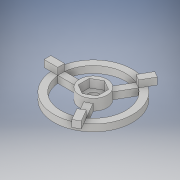
# Autodesk Inventor part: Screw
Saved by Autodesk Inventor 2019 (Build 230136000, 136)
## iProperties
Created: 2018-06-22
Part Number: Screw
Material: Ogólny
Document SubType Name: Modeling
Designer: Kamil
Density: 1 g/cm^3
Appearance: Domyślna
Author: Kamil
Autodesk Inventor part; units mm, degrees
ref_plane "YZ Plane" through (0, 0, 0) normal (1, 0, 0) x (0, 1, 0)
ref_plane "XZ Plane" through (0, 0, 0) normal (0, 1, 0) x (-1, 0, 0)
ref_plane "XY Plane" through (0, 0, 0) normal (0, 0, 1) x (1, 0, 0)
sketch "Szkic1" plane through (0, 0, 0) normal (0, 1, 0) x (-1, 0, 0)
  circle A0 centre (0, 0) radius 28.5
  line L0 (7, -4.0415) -> (0, -8.0829)
  line L1 (0, -8.0829) -> (-1.3414, -7.3085)
  line L2 (-7, -4.0415) -> (-7, 4.0415)
  line L3 (-7, 4.0415) -> (-5.9094, 4.6711)
  line L4 (0, 8.0829) -> (7, 4.0415)
  line L5 (7, 4.0415) -> (7, 2.5)
  line L6 (-1.3414, 7.3085) -> (15.0261, 7.3085) construction
  line L7 (-5.9094, 4.6711) -> (10.4253, 4.6711) construction
  line L8 (-5.9094, -4.6711) -> (10.4253, -4.6711) construction
  line L9 (-1.2173, -7.3801) -> (15.1344, -7.3801) construction
  line L10 (-5.6799, 4.8036) -> (10.6849, 4.8036) construction
  line L11 (-1.3414, -7.3085) -> (-1.3827, -7.3801)
  line L12 (-1.3414, -7.3085) -> (15.0261, -7.3085) construction
  line L13 (-5.6799, -4.8036) -> (10.6849, -4.8036) construction
  arc A1 (23.3666, 2.5) -> (-9.5251, 21.4831) centre (0, 0) ccw
  arc A2 (23.3666, -2.5) -> (23.3666, 2.5) centre (0, 0) ccw
  line L14 (7, -2.5) -> (7, -4.0415)
  line L15 (7, 2.5) -> (7, -2.5)
  line L16 (-1.3414, -7.3085) -> (-5.6799, -4.8036)
  line L17 (-5.6799, -4.8036) -> (-5.9094, -4.6711)
  arc A3 (-9.5251, -21.4831) -> (23.3666, -2.5) centre (0, 0) ccw
  arc A4 (-13.8623, -18.976) -> (-9.5251, -21.4831) centre (0, 0) ccw
  line L18 (-1.3414, 7.3085) -> (0, 8.0829)
  line L19 (-2.6835, 9.6332) -> (-9.5251, 21.4831)
  line L20 (-7.0189, 7.1229) -> (-13.8623, 18.976)
  line L21 (-5.9094, 4.6711) -> (-1.3414, 7.3085)
  line L22 (9.6825, 2.5) -> (23.3666, 2.5)
  arc A5 (8.842, -4.6711) -> (9.6825, -2.5) centre (0, 0) ccw
  line L23 (-2.6835, -9.6332) -> (-9.5251, -21.4831)
  arc A6 (-13.8623, 18.976) -> (-13.8623, -18.976) centre (0, 0) ccw
  line L24 (-7.0189, -7.1229) -> (-7.1674, -7.3801)
  line L25 (-7, -7.0902) -> (-7.0189, -7.1229)
  arc A7 (-2.6835, -9.6332) -> (8.842, -4.6711) centre (0, 0) ccw
  line L26 (-5.9094, -4.6711) -> (-7, -4.0415)
  arc A8 (-7.0189, 7.1229) -> (-7.0189, -7.1229) centre (0, 0) ccw
  line L27 (-7.1674, -7.3801) -> (-13.8623, -18.976)
  arc A9 (-2.6847, -9.6329) -> (-2.6835, -9.6332) centre (0, 0) ccw
  line L28 (9.6825, -2.5) -> (23.3666, -2.5)
  arc A10 (9.6825, 2.5) -> (-2.6835, 9.6332) centre (0, 0) ccw
  line L29 (9.6699, -2.5) -> (9.6825, -2.5)
  point P0 (7, 0)
  point P1 (-13.8623, 18.976)
  point P2 (-13.8623, 18.976)
  dimension "d0" = 57
  constraints: 60 end point, 32 point on circle, 22 coincident, 12 point on line, 11 centre point, 9 horizontal, 2 parallel, 13 other
  measures "d0" diameter of A0
extrude "Wyciągnięcie proste1" add sketch "Szkic1" along normal blind 5 contours A0 | A2 L28 A9 L22 | A9 A5 A7 A8 | A4 L27 L24 A9 L23
sketch "Szkic2" plane through (0, 5, 0) normal (0, 1, 0) x (1, 0, 0)
  line L0 (9.5252, -21.4833) -> (13.8623, -18.9761)
  line L1 (13.8623, -18.9761) -> (18.8672, -27.6335)
  line L2 (18.8672, -27.6335) -> (14.53, -30.1408)
  line L3 (14.53, -30.1408) -> (9.5252, -21.4833)
  line L4 (13.8623, 18.9761) -> (9.5252, 21.4835)
  line L5 (9.5252, 21.4835) -> (14.5304, 30.1408)
  line L6 (14.5304, 30.1408) -> (18.8675, 27.6333)
  line L7 (18.8675, 27.6333) -> (13.8623, 18.9761)
  line L8 (-23.3679, -2.497) -> (-23.3679, 2.4994)
  line L9 (-23.3679, 2.4994) -> (-33.3679, 2.4994)
  line L10 (-33.3679, 2.4994) -> (-33.3679, -2.497)
  line L11 (-33.3679, -2.497) -> (-23.3679, -2.497)
  point P0 (0, 0)
  dimension "d14" = 10
  dimension "d15" = 10
  dimension "d16" = 10
  constraints: 24 end point, 6 parallel, 3 perpendicular, 1 vertical
  measures "d14" distance of L0.end L1.end
  measures "d15" distance of L4.end L5.end
  measures "d16" distance of L9.end L8.end
extrude "Wyciągnięcie proste2" add sketch "Szkic2" along normal blind 5
sketch "Szkic3" plane through (0, 0, 0) normal (0, -1, 0) x (1, 0, 0)
  line L0 (7, -4.0415) -> (0, -8.0829)
  line L1 (0, -8.0829) -> (-7, -4.0415)
  line L2 (-7, -4.0415) -> (-7, 4.0415)
  line L3 (-7, 4.0415) -> (0, 8.0829)
  line L4 (0, 8.0829) -> (7, 4.0415)
  line L5 (7, 4.0415) -> (7, -4.0415)
  circle A0 centre (0, 0) radius 4
  point P0 (7, 0)
  dimension "d19" = 8
  constraints: 12 end point, 2 coincident, 1 centre point, 1 midpoint, 13 other
  measures "d19" diameter of A0
extrude "Wyciągnięcie proste3" add sketch "Szkic3" against normal blind 2
sketch "Szkic4" plane through (0, 5, 0) normal (0, 1, 0) x (1, 0, 0)
  circle A0 centre (0, 0) radius 10
  line L0 (-7, 4.0415) -> (0, 8.0829)
  line L1 (0, 8.0829) -> (7, 4.0415)
  line L2 (7, 4.0415) -> (7, -4.0415)
  line L3 (7, -4.0415) -> (0, -8.0829)
  line L4 (0, -8.0829) -> (-7, -4.0415)
  line L5 (-7, -4.0415) -> (-7, 4.0415)
  point P0 (-7, 0)
  dimension "d22" = 20
  constraints: 12 end point, 2 coincident, 1 centre point, 1 midpoint, 13 other
  measures "d22" diameter of A0
extrude "Wyciągnięcie proste4" add sketch "Szkic4" along normal blind 3
